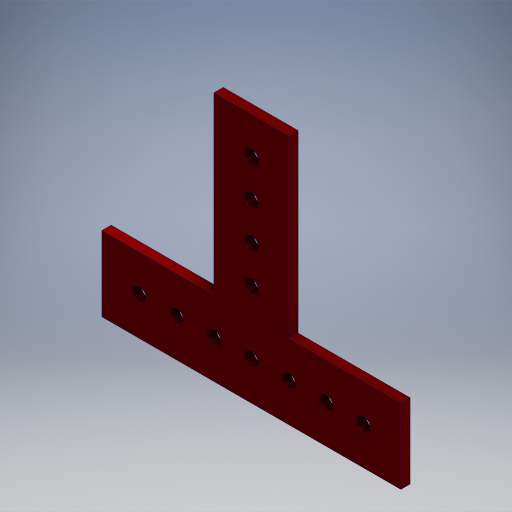
# Autodesk Inventor part: Custom-Underside-T-Gusset
Saved by Autodesk Inventor 2024.2 (Build 282272000, 272)
## iProperties
Created: 2024-02-11
Part Number: Custom-Underside-T-Gusset
Material: Aluminum 6061
Document SubType Name: Modeling
Designer: rohan
Density: 2.7 g/cm^3
Appearance: Aluminum - Flat
Author: rohan
Autodesk Inventor part; units mm, degrees
ref_plane "YZ Plane" through (0, 0, 0) normal (1, 0, 0) x (0, 1, 0)
ref_plane "XZ Plane" through (0, 0, 0) normal (0, 1, 0) x (-1, 0, 0)
ref_plane "XY Plane" through (0, 0, 0) normal (0, 0, 1) x (1, 0, 0)
sketch "Sketch1" plane through (0, 0, 0) normal (0, 0, 1) x (1, 0, 0)
  circle A0 centre (0, 0) radius 2.4892
  circle A1 centre (0, 21.4884) radius 2.4892
  line L0 (-15.227, -8.5114) -> (-2.527, -8.5114) construction
  line L1 (-8.877, -8.5114) -> (-8.877, -14.8614) construction
  circle A2 centre (12.7, 0) radius 2.4892
  circle A3 centre (25.4, 0) radius 2.4892
  circle A4 centre (38.1, 0) radius 2.4892
  circle A5 centre (-12.7, 0) radius 2.4892
  circle A6 centre (-25.4, 0) radius 2.4892
  circle A7 centre (-38.1, 0) radius 2.4892
  circle A8 centre (0, 34.1884) radius 2.4892
  circle A9 centre (0, 46.8884) radius 2.4892
  circle A10 centre (0, 59.5884) radius 2.4892
  line L2 (50.8, 12.7) -> (50.8, -12.7)
  line L3 (50.8, -12.7) -> (-50.8, -12.7)
  line L4 (-50.8, -12.7) -> (-50.8, 12.7)
  line L5 (-12.7, 72.2884) -> (12.7, 72.2884)
  line L6 (12.7, 72.2884) -> (12.7, 12.7)
  line L7 (-8.877, 12.7) -> (-12.7, 12.7)
  line L8 (-12.7, 12.7) -> (-12.7, 72.2884)
  line L9 (-50.8, 12.7) -> (-12.7, 12.7)
  line L10 (12.7, 12.7) -> (50.8, 12.7)
  dimension "d0" = 4.9784
  dimension "d1" = 4.9784
  dimension "d2" = 21.4884
  dimension "d3" = 12.7
  dimension "d4" = 6.35
  dimension "d7" = 12.7
  dimension "d14" = 12.7
  dimension "d21" = 12.7
  dimension "d33" = 25.4
  constraints: 22 end point, 11 centre point, 6 horizontal, 5 parallel, 3 perpendicular, 2 vertical, 1 coincident, 1 midpoint, 1 point on line, 18 other
  measures "d0" diameter of A0
  measures "d1" diameter of A1
  measures "d2" distance of point (0, 0) A1.centre
  measures "d3" distance of L0.start L0.end
  measures "d4" distance of L1.start L1.end
  measures "d7" distance of A0.centre A2.centre
  measures "d14" distance of A0.centre A5.centre
  measures "d21" distance of A1.centre A8.centre
  measures "d33" distance of L6.end L7.end
extrude "Extrusion1" add sketch "Sketch1" along normal blind 3.175
body "Solid1"
